# Autodesk Inventor part: CSTCR4M00G15L99
Saved by Autodesk Inventor 2016 SP1 (Build 200210100, 210)
## iProperties
Created: 2015-11-24
Part Number: CSTCR4M00G15L99
Material: Generic
Document SubType Name: Modeling
Designer: PhillipD
Density: 1 g/cm^3
Appearance: MURATA-FILTER_CSTCR, CSTCR4M00G15L99
Author: PhillipD
Autodesk Inventor part; units mm, degrees
ref_plane "YZ Plane" through (0, 0, 0) normal (1, 0, 0) x (0, 1, 0)
ref_plane "XZ Plane" through (0, 0, 0) normal (0, 1, 0) x (-1, 0, 0)
ref_plane "XY Plane" through (0, 0, 0) normal (0, 0, 1) x (1, 0, 0)
sketch "MURATA-FILTER_CSTCR, CSTCR4M00G15L99_93" plane through (0, 0, 0) normal (0, 0, 1) x (1, 0, 0)
  line L0 (-2.2508, 1.4) -> (2.2508, 1.4)
  line L1 (2.2508, 1.4) -> (2.2508, -1.4)
  line L2 (2.2508, -1.4) -> (-2.2508, -1.4)
  line L3 (-2.2508, -1.4) -> (-2.2508, 1.4)
  constraints: 8 end point
extrude "Extrusion1" add sketch "MURATA-FILTER_CSTCR, CSTCR4M00G15L99_93" along normal blind 1
body "Solid1"
